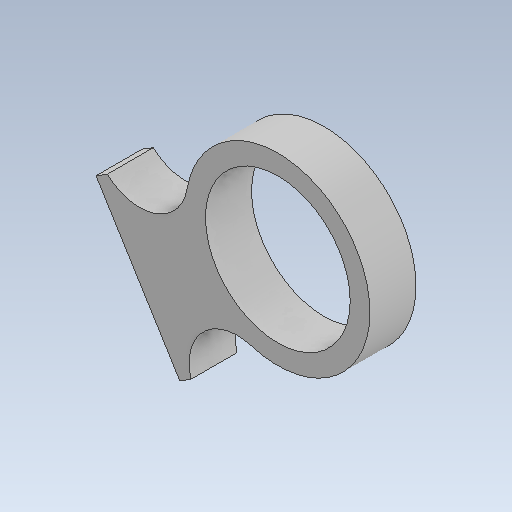
# Autodesk Inventor part: SoportePolea
Saved by Autodesk Inventor 2021 (Build 250183000, 183)
## iProperties
Created: 2022-10-28
Part Number: SoportePolea
Material: Generic
Document SubType Name: Modeling
Designer: zulet
Density: 1 g/cm^3
Appearance: Default
Author: zulet
Autodesk Inventor part; units mm, degrees
ref_plane "YZ Plane" through (0, 0, 0) normal (1, 0, 0) x (0, 1, 0)
ref_plane "XZ Plane" through (0, 0, 0) normal (0, 1, 0) x (-1, 0, 0)
ref_plane "XY Plane" through (0, 0, 0) normal (0, 0, 1) x (1, 0, 0)
sketch "Sketch1" plane through (0, 0, 0) normal (0, 0, 1) x (1, 0, 0)
  circle A0 centre (0, 0) radius 4
  circle A1 centre (0, 0) radius 11
  arc A2 (-4.0518, -13.4009) -> (-13.7956, 2.3837) centre (0, 0) ccw
  line L0 (-25.9378, -1.7681) -> (-27.6396, -2.8187) projected
  line L1 (-27.6396, -2.8187) -> (-14.9069, -23.4452) projected
  line L2 (-14.9069, -23.4452) -> (-13.205, -22.3947) projected
  arc A3 (-25.9378, -1.7681) -> (-13.7956, 2.3837) centre (-21.0023, 3.6289) ccw
  line L3 (0, 0) -> (11.913, 7.3539) construction
  arc A4 (-4.0518, -13.4009) -> (-13.205, -22.3947) centre (-6.1684, -20.4014) ccw
  dimension "d0" = 8
  dimension "d1" = 22
  dimension "d2" = 3
  dimension "d3" = 2
  constraints: 7 point on circle, 5 centre point, 2 coincident, 2 end point, 2 symmetric about line, 1 perpendicular, 1 tangent, 1 other
  measures "d0" diameter of A0
  measures "d1" diameter of A1
  measures "d2" radial gap between concentric circles of A1 A2
  measures "d3" distance from line of L0 A3.centre
extrude "Extrusion1" add sketch "Sketch1" along normal blind 7 contours A4 L2 L1 L0 A3 A2
equation "\"d0\" = DIR"
equation "\"d1\" = DER"
equation "\"d2\" = TB"
equation "\"DER\" = 22"
equation "\"HR\" = 7"
equation "\"DIR\" = 8"
equation "\"DEM\" = 4"
equation "\"Dmarc\" = 17.5"
equation "\"Bsm\" = 22.5"
equation "\"Hsm\" = 12"
equation "\"Lsm\" = 21"
equation "\"Dsc\" = 5"
equation "\"RC\" = 4"
equation "\"PB\" = 25"
equation "\"TB\" = 3"
equation "\"HSE\" = 25"
body "Solid1"
